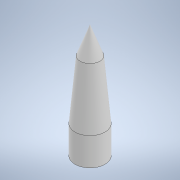
# Autodesk Inventor part: nockForCalli
Saved by Autodesk Inventor 2021.1 (Build 251245010, 245A)
## iProperties
Created: 2020-11-04
Part Number: nockForCalli
Material: Generic
Document SubType Name: Modeling
Designer: robst
Density: 1 g/cm^3
Appearance: Default
Author: robst
Autodesk Inventor part; units mm, degrees
ref_plane "YZ Plane" through (0, 0, 0) normal (1, 0, 0) x (0, 1, 0)
ref_plane "XZ Plane" through (0, 0, 0) normal (0, 1, 0) x (-1, 0, 0)
ref_plane "XY Plane" through (0, 0, 0) normal (0, 0, 1) x (1, 0, 0)
sketch "Sketch2" plane through (0, 0, 0) normal (0, 0, 1) x (1, 0, 0)
  line L0 (0, 0) -> (5.334, 0) construction
  line L1 (5.334, 0) -> (5.334, 40.3652) construction
  line L2 (5.334, 40.3652) -> (0, 40.3652) construction
  line L3 (0, 40.3652) -> (0, 0) construction
  line L4 (4.064, 0) -> (4.064, 9.525)
  line L5 (4.064, 9.525) -> (2.2844, 30.3887)
  line L6 (0, 31.115) -> (1.4936, 31.115) construction
  line L7 (0, 9.525) -> (4.064, 9.525) construction
  line L8 (5.334, 0) -> (5.334, 9.9113)
  line L9 (5.334, 9.9113) -> (3.4925, 30.7697)
  line L10 (0, 31.115) -> (2.2225, 31.115)
  line L11 (3.4925, 30.7697) -> (0, 40.3652)
  line L12 (4.064, 0) -> (5.334, 0)
  line L13 (0, 40.3652) -> (0, 31.115)
  arc A0 (2.2844, 30.3887) -> (1.4936, 31.115) centre (1.4936, 30.3212) ccw
  dimension "d6" = 5.334
  dimension "d7" = 4.064
  dimension "d8" = 21.59
  dimension "d9" = 2.2225
  dimension "d10" = 9.525
  dimension "d11" = 1.27
  dimension "d13" = 20
  dimension "d14" = 0.7937
  constraints: 28 end point, 6 point on line, 3 horizontal, 2 collinear, 2 parallel, 2 perpendicular, 2 point on circle, 2 tangent, 1 centre point, 1 equal length, 1 vertical
  measures "d6" distance between parallel lines of L1 L3
  measures "d7" distance between parallel lines of L4 L3
  measures "d8" distance between parallel lines of L7 L6
  measures "d9" distance from line of L10.end L3
  measures "d10" distance between parallel lines of L7 L0
  measures "d11" horizontal distance of L9.end L10.end
  measures "d13" angle of L11 L3
  measures "d14" radius of A0
revolve "Revolution1" add sketch "Sketch2" angle 360 about axis through (0, 40.3652, 0) along (0, -1, 0)
equation "\"d6\" = shaftRadius + arrowWallThickness"
equation "\"d7\" = shaftRadius"
equation "\"d8\" = shaftAngledLength"
equation "\"d9\" = shaftTipRadius"
equation "\"d11\" = arrowWallThickness"
equation "\"shaftTipDiameter\" = 4.445"
equation "\"shaftDiameter\" = 8.128"
equation "\"shaftAngledLength\" = 21.59"
equation "\"arrowTotalLength\" = 31.75"
equation "\"shaftTipRadius\" = 0.5 * shaftTipDiameter"
equation "\"shaftRadius\" = 0.5 * shaftDiameter"
equation "\"arrowWallThickness\" = 1.27"
body "Solid1"
